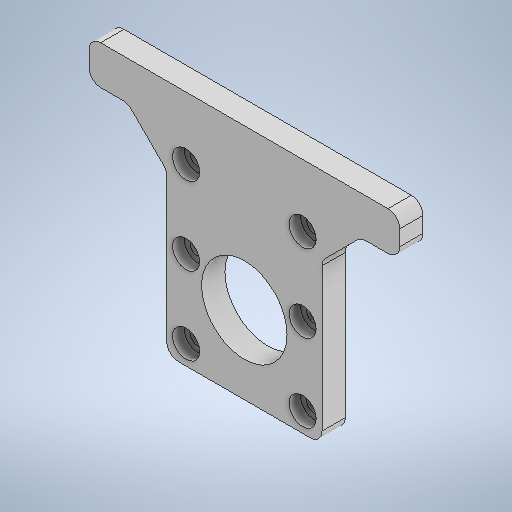
# Autodesk Inventor part: stopper_motor_bracket_cover
Saved by Autodesk Inventor 2026.1 (Build 301233000, 233)
## iProperties
Created: 2026-05-21
Part Number: stopper_motor_bracket_cover
Material: Generic
Document SubType Name: Modeling
Designer: chris
Density: 1 g/cm^3
Appearance: Default
Author: chris
Autodesk Inventor part; units mm, degrees
ref_plane "YZ Plane" through (0, 0, 0) normal (1, 0, 0) x (0, 1, 0)
ref_plane "XZ Plane" through (0, 0, 0) normal (0, 1, 0) x (-1, 0, 0)
ref_plane "XY Plane" through (0, 0, 0) normal (0, 0, 1) x (1, 0, 0)
sketch "Sketch1" plane through (0, 0, 0) normal (0, 0, 1) x (1, 0, 0)
  line L0 (-40, -40) -> (40, -40)
  line L1 (40, -40) -> (40, 40)
  line L2 (40, 40) -> (-40, 40)
  line L3 (-40, 40) -> (-40, -40)
  line L4 (-40, -40) -> (40, 40) construction
  line L5 (40, -40) -> (-40, 40) construction
  point P0 (0, 0)
  dimension "d0" = 80
  dimension "d1" = 80
  constraints: 12 end point, 2 midpoint, 2 parallel, 1 horizontal, 1 perpendicular
  measures "d0" distance of L2.end L1.end
  measures "d1" distance of L1.end L0.end
extrude "Extrusion1" add sketch "Sketch1" along normal blind 6
sketch "Sketch2" plane through (0, 0, 6) normal (0, 0, 1) x (1, 0, 0)
  arc A0 (-37, 21.1) -> (-40, 18.1) centre (-37, 18.1) ccw projected
  line L0 (-40, 14.1) -> (-40, 18.1) projected
  arc A1 (-40, 14.1) -> (-37, 11.1) centre (-37, 14.1) ccw projected
  line L1 (-37, 11.1) -> (-31.2426, 11.1) projected
  arc A2 (-29.1213, 10.2213) -> (-31.2426, 11.1) centre (-31.2426, 8.1) ccw projected
  line L2 (-29.1213, 10.2213) -> (-20.8787, 1.9787) projected
  arc A3 (-20, -0.1426) -> (-20.8787, 1.9787) centre (-23, -0.1426) ccw projected
  line L3 (-20, -0.1426) -> (-20, -37) projected
  arc A4 (-20, -37) -> (-17, -40) centre (-17, -37) ccw projected
  line L4 (-17, -40) -> (17, -40) projected
  arc A5 (17, -40) -> (20, -37) centre (17, -37) ccw projected
  line L5 (20, -37) -> (20, -0.1426) projected
  arc A6 (20.8787, 1.9787) -> (20, -0.1426) centre (23, -0.1426) ccw projected
  line L6 (20.8787, 1.9787) -> (29.1213, 10.2213) projected
  arc A7 (31.2426, 11.1) -> (29.1213, 10.2213) centre (31.2426, 8.1) ccw projected
  line L7 (31.2426, 11.1) -> (37, 11.1) projected
  arc A8 (37, 11.1) -> (40, 14.1) centre (37, 14.1) ccw projected
  line L8 (40, 14.1) -> (40, 18.1) projected
  arc A9 (40, 18.1) -> (37, 21.1) centre (37, 18.1) ccw projected
  line L9 (-37, 21.1) -> (37, 21.1) projected
  line L10 (10.1, -30) -> (10.1, 11.1) projected
  line L11 (10.1, -30) -> (-10.1, -30) projected
  line L12 (-10.1, -30) -> (-10.1, 11.1) projected
  line L13 (-10.1, 11.1) -> (10.1, 11.1) projected
  circle A10 centre (15, -35) radius 2 projected
  circle A11 centre (-15, -15) radius 2 projected
  circle A12 centre (-15, -35) radius 2 projected
  circle A13 centre (15, -15) radius 2 projected
  circle A14 centre (-15, 5) radius 2 projected
  circle A15 centre (15, 5) radius 2 projected
  line L14 (-40, -40) -> (40, -40)
  line L15 (40, -40) -> (40, 40)
  line L16 (40, 40) -> (-40, 40)
  line L17 (-40, 40) -> (-40, -40)
  line L18 (-40, -40) -> (40, 40) construction
  line L19 (40, -40) -> (-40, 40) construction
  line L20 (40, 40) -> (-40, 40) projected
  line L21 (40, -40) -> (40, 40) projected
  line L22 (-10.1, -30) -> (10.1, -30)
  line L23 (10.1, -30) -> (10.1, 11.1)
  line L24 (10.1, 11.1) -> (-10.1, 11.1)
  line L25 (-10.1, 11.1) -> (-10.1, -30)
  line L26 (-10.1, -30) -> (10.1, 11.1) construction
  line L27 (10.1, -30) -> (-10.1, 11.1) construction
  point P0 (0, 0)
  point P1 (40, 14.1)
  point P2 (0, -9.45)
  constraints: 24 end point, 6 collinear, 4 midpoint, 4 parallel, 2 horizontal, 2 perpendicular
sketch "Sketch3" plane through (0, 0, 6) normal (0, 0, 1) x (1, 0, 0)
  line L0 (37, 14.1) -> (37, 21.1) projected
  line L1 (23, 14.1) -> (37, 14.1) projected
  arc A0 (23, 14.1) -> (17, 8.1) centre (23, 8.1) ccw projected
  line L2 (17, -37) -> (17, 8.1) projected
  line L3 (-17, -37) -> (17, -37) projected
  line L4 (-17, 8.1) -> (-17, -37) projected
  arc A1 (-17, 8.1) -> (-23, 14.1) centre (-23, 8.1) ccw projected
  line L5 (-37, 14.1) -> (-23, 14.1) projected
  line L6 (-37, 21.1) -> (-37, 14.1) projected
  line L7 (37, 21.1) -> (-37, 21.1) projected
  circle A2 centre (0, -20) radius 7.5 projected
  circle A3 centre (-7.525, -27.5) radius 2 projected
  circle A4 centre (7.525, -27.5) radius 2 projected
  circle A5 centre (7.525, 7.6) radius 2 projected
  circle A6 centre (-7.525, 7.6) radius 2 projected
  circle A7 centre (7.525, -7.5) radius 2 projected
  circle A8 centre (-7.525, -7.5) radius 2 projected
  circle A9 centre (0, -20) radius 11
  point P0 (0, 0)
  dimension "d4" = 22
  constraints: 1 centre point, 1 coincident
  measures "d4" diameter of A9
extrude "Extrusion2" cut sketch "Sketch2" against normal blind 7 contours A0 L17 L16 L15 A9 L9 | A1 L1 A2 L2 A3 L3 A4 L14 L17 | L15 L14 A5 L5 A6 L6 A7 L7 A8 | A10 | A11 | A12 | A13 | A14 | A15
extrude "Extrusion3" cut sketch "Sketch3" against normal blind 7 contours A2 | A3 A9 | A3 A9 A4 | A4 A9 picked at (-7.1985, -27.22) picked at (7.2207, -27.1967)
sketch "Sketch4" plane through (0, 0, 6) normal (0, 0, 1) x (1, 0, 0)
  circle A0 centre (-15, 5) radius 2 projected
  circle A1 centre (15, 5) radius 2 projected
  circle A2 centre (-15, -15) radius 2 projected
  circle A3 centre (15, -15) radius 2 projected
  circle A4 centre (-15, -35) radius 2 projected
  circle A5 centre (15, -35) radius 2 projected
  circle A6 centre (15, 5) radius 3.5
  circle A7 centre (15, -15) radius 3.5
  circle A8 centre (15, -35) radius 3.5
  circle A9 centre (-15, -35) radius 3.5
  circle A10 centre (-15, -15) radius 3.5
  circle A11 centre (-15, 5) radius 3.5
  point P0 (0, 0)
  dimension "d9" = 7
  dimension "d10" = 7
  dimension "d11" = 7
  dimension "d12" = 7
  dimension "d13" = 7
  dimension "d14" = 7
  constraints: 6 centre point, 6 coincident
  measures "d9" diameter of A6
  measures "d10" diameter of A7
  measures "d11" diameter of A8
  measures "d12" diameter of A9
  measures "d13" diameter of A10
  measures "d14" diameter of A11
extrude "Extrusion4" cut sketch "Sketch4" against normal blind 3
body "Solid1"
